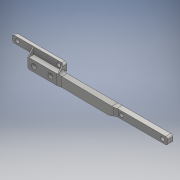
# Autodesk Inventor part: PanTiltMount
Saved by Autodesk Inventor 2016 (Build 200138000, 138)
## iProperties
Created: 2026-02-03
Part Number: PanTiltMount
Material: Generic
Document SubType Name: Modeling
Designer: Steve
Density: 1 g/cm^3
Appearance: Default
Author: Steve
Autodesk Inventor part; units mm, degrees
ref_plane "YZ Plane" through (0, 0, 0) normal (1, 0, 0) x (0, 1, 0)
ref_plane "XZ Plane" through (0, 0, 0) normal (0, 1, 0) x (-1, 0, 0)
ref_plane "XY Plane" through (0, 0, 0) normal (0, 0, 1) x (1, 0, 0)
sketch "Sketch1" plane through (0, 0, 0) normal (0, 1, 0) x (-1, 0, 0)
  line L0 (30, 0) -> (30, -10)
  line L1 (30, -10) -> (-1.0657, -10)
  line L2 (-1.0657, -10) -> (-27.4657, -32)
  line L3 (-27.4657, -32) -> (-81, -32)
  line L4 (-81, -32) -> (-81, -25)
  line L5 (-81, -25) -> (-30, -25)
  line L6 (-30, -25) -> (0, 0)
  circle A0 centre (24, -5) radius 2.25
  circle A1 centre (8, -5) radius 2.25
  circle A2 centre (-76, -28.5) radius 1.75
  circle A3 centre (-36, -28.5) radius 1.75
  line L7 (0, 0) -> (0, 0)
  line L8 (0, 0) -> (0, 6.6)
  line L9 (0, 6.6) -> (50, 6.6)
  line L10 (50, 6.6) -> (50, 0)
  line L11 (50, 0) -> (30, 0)
  circle A4 centre (5, 3.3) radius 1.75
  circle A5 centre (45, 3.3) radius 1.75
  dimension "d0" = 10
  dimension "d1" = 7
  dimension "d2" = 7
  dimension "d3" = 30
  dimension "d6" = 25
  dimension "d7" = 30
  dimension "d8" = 4.5
  dimension "d9" = 4.5
  dimension "d10" = 5
  dimension "d11" = 5
  dimension "d12" = 6
  dimension "d13" = 16
  dimension "d14" = 3.5
  dimension "d15" = 5
  dimension "d16" = 3.5
  dimension "d17" = 3.5
  dimension "d18" = 3.5
  dimension "d19" = 40
  dimension "d20" = 51
  dimension "d21" = 50
  dimension "d22" = 6.6
  dimension "d23" = 20
  dimension "d24" = 3.5
  dimension "d25" = 8.3
  dimension "d26" = 3.5
  dimension "d27" = 40
  dimension "d28" = 5
  dimension "d29" = 8.3
  constraints: 24 end point, 7 perpendicular, 6 centre point, 2 parallel, 1 horizontal, 1 point on line, 1 vertical
  measures "d0" distance of L0.start L0.end
  measures "d1" distance of L3.end L4.end
  measures "d2" distance between parallel lines of L2 L6
  measures "d3" distance of L0.start L6.end
  measures "d6" vertical distance of L6.end L4.end
  measures "d7" horizontal distance of L6.end L5.end
  measures "d8" diameter of A0
  measures "d9" diameter of A1
  measures "d10" distance from line of L1 A0.centre
  measures "d11" distance from line of L1 A1.centre
  measures "d12" distance from line of L0 A0.centre
  measures "d13" distance of A0.centre A1.centre
  measures "d14" diameter of A2
  measures "d15" distance from line of L4 A2.centre
  measures "d16" diameter of A3
  measures "d17" distance from line of L3 A3.centre
  measures "d18" distance from line of L3 A2.centre
  measures "d19" distance of A3.centre A2.centre
  measures "d20" distance of L4.end L5.end
  measures "d21" distance of L8.end L9.end
  measures "d22" distance of L7.end L8.end
  measures "d23" distance of L10.end L0.start
  measures "d24" diameter of A4
  measures "d25" vertical distance of A1.centre A4.centre
  measures "d26" diameter of A5
  measures "d27" distance of A4.centre A5.centre
  measures "d28" distance from line of L10 A5.centre
  measures "d29" vertical distance of A5.centre A0.centre
extrude "Extrusion1" add sketch "Sketch1" along normal blind 30
sketch "Sketch8" plane through (0, 30, 0) normal (0, 1, 0) x (1, 0, 0)
  line L0 (1.0657, 10) -> (-30, 10) projected
  line L1 (-30, 10) -> (0, 10)
  line L2 (0, 10) -> (0, 2)
  line L3 (0, 2) -> (-30, 2)
  line L4 (-30, 2) -> (-30, 10)
  circle A0 centre (-8, 5) radius 2.25 projected
  point P0 (0, 0)
  dimension "d41" = 3
  constraints: 8 end point, 2 parallel, 1 horizontal, 1 perpendicular
  measures "d41" distance from line of L3 A0.centre
extrude "Extrusion5" cut sketch "Sketch8" against normal blind 25
sketch "Sketch12" plane through (0, 0, 0) normal (0, -1, 0) x (1, 0, 0)
  line L0 (-50, 0) -> (-50, 6.6) projected
  line L1 (-50, 6.6) -> (0, 6.6)
  line L2 (0, 6.6) -> (0, 0)
  line L3 (0, 0) -> (-50, 0)
  line L4 (-50, 0) -> (-50, 6.6)
  constraints: 8 end point, 2 parallel, 1 horizontal, 1 perpendicular
extrude "Extrusion6" cut sketch "Sketch12" against normal blind 5
sketch "Sketch13" plane through (0, 30, 0) normal (0, 1, 0) x (1, 0, 0)
  line L0 (-50, -6.6) -> (0, -6.6) projected
  line L1 (-50, 0) -> (-50, -6.6) projected
  line L2 (0, -6.6) -> (-50, -6.6)
  line L3 (-50, -6.6) -> (-50, 0)
  line L4 (-30, 0) -> (-50, 0) projected
  line L5 (-50, 0) -> (-30, 0)
  line L6 (-30, 2) -> (-30, 0) projected
  line L7 (-30, 0) -> (-30, 2)
  line L8 (0, 2) -> (-30, 2) projected
  line L9 (-30, 2) -> (0, 2)
  line L10 (0, 2) -> (0, -6.6)
  point P0 (0, 0)
  constraints: 12 end point, 2 collinear, 2 perpendicular, 1 horizontal, 1 vertical
extrude "Extrusion7" cut sketch "Sketch13" against normal blind 22
sketch "Sketch19" plane through (0, 0, 0) normal (0, 0, 1) x (1, 0, 0)
  line L0 (81, 0) -> (81, 30) projected
  line L1 (81, 30) -> (81, 25)
  line L2 (81, 25) -> (31, 25)
  line L3 (30, 0) -> (30, 30) projected
  line L4 (30, 0) -> (81, 0) projected
  line L5 (0, 0) -> (81, 0)
  line L6 (81, 0) -> (81, 25)
  line L7 (0, 0) -> (31, 25)
  dimension "d59" = 5
  dimension "d60" = 50
  dimension "d61" = 90
  constraints: 10 end point, 3 perpendicular, 1 point on line
  measures "d59" distance of L0.end L1.end
  measures "d60" distance of L1.end L2.end
  measures "d61" angle of L1 L2
extrude "Extrusion9" cut sketch "Sketch19" against normal blind 50
sketch "Sketch20" plane through (0, 0, 0) normal (0, 0, 1) x (1, 0, 0)
  line L0 (0, 5) -> (0, 8) projected
  line L1 (30, 24.1935) -> (30, 30) projected
  line L2 (0, 5) -> (30, 30)
  line L3 (1.0657, 30) -> (0, 30) projected
  line L4 (30, 30) -> (0, 30)
  line L5 (0, 30) -> (0, 5)
  point P0 (0, 0)
  point P1 (30, 25)
  constraints: 6 end point, 1 collinear, 1 perpendicular
extrude "Extrusion10" cut sketch "Sketch20" against normal blind 50
sketch "Sketch24" plane through (0, 5, 6.6) normal (1, 0, 0) x (0, 0, -1)
  line L0 (6.6, -5) -> (6.6, 0) projected
  line L1 (6.6, 0) -> (6.6, -5)
  line L2 (6.6, -5) -> (0, 0)
  line L3 (0, 0) -> (6.6, 0)
  constraints: 6 end point, 1 collinear, 1 perpendicular
extrude "Extrusion11" add sketch "Sketch24" against normal blind 1
sketch "Sketch25" plane through (-30, 0, -10) normal (-1, 0, 0) x (0, 0, 1)
  line L0 (10, 5.0528) -> (10, 0)
  line L1 (10, 0) -> (16.5609, 5)
  line L2 (10, 0) -> (10, 5) projected
  line L3 (16.5609, 5) -> (10, 5)
  constraints: 6 end point, 1 perpendicular, 1 vertical
extrude "Extrusion12" add sketch "Sketch25" against normal blind 1
fillet "Fillet37" radius 5 4 edges at (27.4657, 25.0189, -32) (30, 30, -28.5) (30, 27.0968, -25) (31, 25, -28.5)
fillet "Fillet38" radius 5 1 edges at (1.0657, 3.3737, -10)
fillet "Fillet39" radius 5 1 edges at (0, 2.5, 0)
fillet "Fillet41" radius 5 1 edges at (0, 5, -6.0279)
fillet "Fillet42" radius 5 1 edges at (0, 0, -5.0279)
fillet "Fillet44" radius 2 3 edges at (-30, 6.5, 0) (-30, 6.5, -2) (0, 6.6696, -2)
fillet "Fillet45" radius 2 1 edges at (-30, 2.5, -10)
fillet "Fillet46" radius 2 5 edges at (-50, 6.5, 0) (-50, 6.5, 6.6) (0, 6.5, 6.6) (81, 27.5, -25) (81, 27.5, -32)
sketch "Sketch26" plane through (0, 5, 0) normal (0, 1, 0) x (1, 0, 0)
  circle A0 centre (-24, 5) radius 2.25 projected
  circle A1 centre (-24, 5) radius 4
  circle A2 centre (-8, 5) radius 4
  point P0 (0, 0)
  dimension "d117" = 8
  dimension "d118" = 8
  dimension "d119" = 16
  constraints: 2 centre point, 1 coincident
  measures "d117" diameter of A1
  measures "d118" diameter of A2
  measures "d119" distance of A2.centre A1.centre
extrude "Extrusion13" cut sketch "Sketch26" along normal blind 3 and the other way blind 2
body "Solid1"
